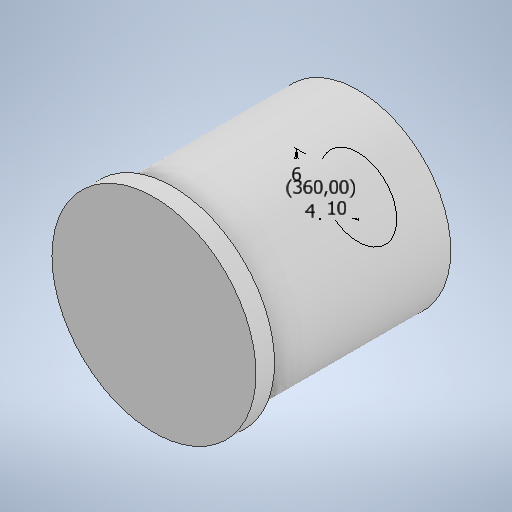
# Autodesk Inventor part: 13042026-03
Saved by Autodesk Inventor 2025.2 (Build 292293000, 293)
## iProperties
Created: 2026-04-14
Part Number: 13042026-03
Material: Generic
Document SubType Name: Modeling
Designer: Oski
Density: 1 g/cm^3
Appearance: Default
Author: Oski
Autodesk Inventor part; units mm, degrees
ref_plane "YZ Plane" through (0, 0, 0) normal (1, 0, 0) x (0, 1, 0)
ref_plane "XZ Plane" through (0, 0, 0) normal (0, 1, 0) x (-1, 0, 0)
ref_plane "XY Plane" through (0, 0, 0) normal (0, 0, 1) x (1, 0, 0)
sketch "Sketch1" plane through (0, 0, 0) normal (0, 0, 1) x (1, 0, 0)
  circle A0 centre (0, 0) radius 25
  dimension "d0" = 50
  constraints: 1 centre point, 1 coincident
  measures "d0" diameter of A0
extrude "Extrusion1" add sketch "Sketch1" along normal blind 50
sketch "Sketch2" plane through (0, 0, 50) normal (0, 0, 1) x (1, 0, 0)
  circle A0 centre (0, 0) radius 27.5
  dimension "d3" = 55
  constraints: 1 centre point, 1 coincident
  measures "d3" diameter of A0
extrude "Extrusion2" add sketch "Sketch2" along normal blind 5
sketch "Sketch3" plane through (0, 0, 0) normal (0, 0, -1) x (-1, 0, 0)
  line L0 (14, 3) -> (10, 3)
  line L1 (10, 3) -> (10, -3)
  line L2 (10, -3) -> (14, -3)
  line L3 (14, -3) -> (14, 3)
  line L4 (10, 0) -> (0, 0) construction
  line L5 (0, 0) -> (0, 3)
  line L6 (0, 0) -> (0, -3)
  line L7 (-2.4019, 10.1603) -> (-4.4019, 13.6244)
  line L8 (-4.4019, 13.6244) -> (-9.5981, 10.6244)
  line L9 (-9.5981, 10.6244) -> (-7.5981, 7.1603)
  line L10 (-7.5981, 7.1603) -> (-2.4019, 10.1603)
  line L11 (-7.5981, -7.1603) -> (-9.5981, -10.6244)
  line L12 (-9.5981, -10.6244) -> (-4.4019, -13.6244)
  line L13 (-4.4019, -13.6244) -> (-2.4019, -10.1603)
  line L14 (-2.4019, -10.1603) -> (-7.5981, -7.1603)
  point P0 (2.5981, 1.5)
  point P1 (-2.5981, -1.5)
  point P2 (-5, 8.6603)
  point P3 (-2.5981, 1.5)
  point P4 (2.5981, -1.5)
  point P5 (-5, -8.6603)
  dimension "d6" = 10
  dimension "d7" = 4
  dimension "d8" = 6
  dimension "d11" = 360
  constraints: 30 end point, 7 point on line, 3 midpoint, 2 horizontal, 2 parallel, 2 perpendicular, 1 collinear, 34 other
  measures "d6" distance of L4.start L4.end
  measures "d7" distance of L1.end L2.end
  measures "d8" distance of L2.end L0.start
body "Solid1"
